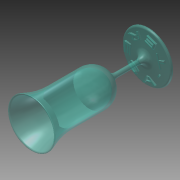
# Autodesk Inventor part: Copas personalizadas
Saved by Autodesk Inventor 2014 (Build 180170000, 170)
## iProperties
Created: 2016-12-26
Part Number: Copas personalizadas
Material: Generic
Document SubType Name: Modeling
Designer: Rubén
Density: 1 g/cm^3
Appearance: Indoor Pool
Author: Rubén
Autodesk Inventor part; units mm, degrees
ref_plane "YZ Plane" through (0, 0, 0) normal (1, 0, 0) x (0, 1, 0)
ref_plane "XZ Plane" through (0, 0, 0) normal (0, 1, 0) x (-1, 0, 0)
ref_plane "XY Plane" through (0, 0, 0) normal (0, 0, 1) x (1, 0, 0)
sketch "Sketch1" plane through (0, 0, 0) normal (1, 0, 0) x (0, 1, 0)
  line L0 (0, 0) -> (0, 70)
  line L1 (0, 70) -> (26, 70)
  line L2 (26, 70) -> (26, 144.9058)
  line L3 (32.0307, 179.1078) -> (36.1508, 190.4275)
  line L4 (38.5, 189.5725) -> (34.38, 178.2528)
  line L5 (28.5, 144.9058) -> (28.5, 67.5)
  line L6 (28.5, 67.5) -> (3.5, 67.5)
  line L7 (3.5, 67.5) -> (3.5, 19.3406)
  line L8 (14.7357, 6.4609) -> (37.4072, 3.3552)
  line L9 (40, 0.3829) -> (40, 0)
  line L10 (40, 0) -> (0, 0)
  line L11 (0, 70) -> (0, 190) construction
  arc A0 (32.0307, 179.1078) -> (26, 144.9058) centre (126, 144.9058) ccw
  arc A1 (34.38, 178.2528) -> (28.5, 144.9058) centre (126, 144.9058) ccw
  line L12 (37.3254, 190) -> (0, 190) construction
  arc A2 (3.5, 19.3406) -> (14.7357, 6.4609) centre (16.5, 19.3406) ccw
  arc A3 (40, 0.3829) -> (37.4072, 3.3552) centre (37, 0.3829) ccw
  line L13 (26, 70) -> (26, 67.5) construction
  line L14 (36.1508, 190.4275) -> (38.5, 189.5725)
  point P0 (26, 162.5385)
  point P1 (28.5, 162.0977)
  point P2 (3.5, 8)
  point P3 (40, 3)
  dimension "d2" = 3
  dimension "d4" = 70
  dimension "d5" = 40
  dimension "d6" = 8
  dimension "d7" = 3.5
  dimension "d10" = 100
  dimension "d14" = 13
  dimension "d15" = 3
  dimension "d26" = 2.5
  dimension "d27" = 10
  dimension "d28" = 26
  dimension "d29" = 160
  dimension "d30" = 190
  constraints: 30 end point, 9 point on line, 8 point on circle, 8 tangent, 5 parallel, 5 perpendicular, 4 centre point, 1 coincident, 1 equal length, 1 horizontal, 1 midpoint, 1 vertical
  measures "d2" distance of point (40, 3) L9.end
  measures "d4" distance of L0.start L0.end
  measures "d5" distance of L9.end L0.start
  measures "d6" distance from line of L10 point (3.5, 8)
  measures "d7" distance between parallel lines of L7 L0
  measures "d10" radius of A0
  measures "d14" radius of A2
  measures "d15" radius of A3
  measures "d26" distance of L1.end L13.end
  measures "d27" distance from line of L5 L4.start
  measures "d28" distance of L0.end L1.end
  measures "d29" angle of L5 L4
  measures "d30" distance between parallel lines of L10 L12
revolve "Revolution1" add sketch "Sketch1" angle 360 about axis through (0, 0, 0) along (0, 0, 1)
fillet "Fillet1" radius 2 2 edges at (0, -36.1508, 190.4275) (0, -38.5, 189.5725)
fillet "Fillet2" radius 26 1 edges at (0, -26, 70)
fillet "Fillet3" radius 15 1 edges at (0, -3.5, 67.5)
fillet "Fillet4" radius 28 1 edges at (0, -28.5, 67.5)
sketch "Sketch2" plane through (0, 0, 0) normal (0, 0, -1) x (-1, 0, 0)
  circle A0 centre (0, 0) radius 40 projected
  constraints: 1 other
extrude "Antonio" [suppressed]
sketch "Sketch3" plane through (0, 0, 0) normal (0, 0, -1) x (-1, 0, 0)
  circle A0 centre (0, 0) radius 40
  line L0 (-32.0557, 8.0153) -> (-23.6218, 5.4451)
  line L1 (-23.6218, 5.4451) -> (-26.0692, -2.5857)
  line L2 (-26.0692, -2.5857) -> (-24.9374, -2.9306)
  line L3 (-24.9374, -2.9306) -> (-19.0741, 16.3092)
  line L4 (-19.0741, 16.3092) -> (-20.2059, 16.6541)
  line L5 (-20.2059, 16.6541) -> (-22.6532, 8.6233)
  line L6 (-22.6532, 8.6233) -> (-31.0872, 11.1935)
  line L7 (-31.0872, 11.1935) -> (-32.0557, 8.0153)
  line L8 (-18.1111, 28.4868) -> (-14.6428, 19.1075)
  line L9 (-14.6428, 19.1075) -> (0.0114, 24.5263)
  line L10 (0.0114, 24.5263) -> (-0.399, 25.636)
  line L11 (-0.399, 25.636) -> (-11.9369, 21.3695)
  line L12 (-11.9369, 21.3695) -> (-12.8869, 23.9386)
  line L13 (-12.8869, 23.9386) -> (-2.1394, 27.9128)
  line L14 (-2.1394, 27.9128) -> (-2.5498, 29.0225)
  line L15 (-2.5498, 29.0225) -> (-13.2972, 25.0483)
  line L16 (-13.2972, 25.0483) -> (-14.5845, 28.5294)
  line L17 (-14.5845, 28.5294) -> (-3.0466, 32.7959)
  line L18 (-3.0466, 32.7959) -> (-3.4569, 33.9056)
  line L19 (-3.4569, 33.9056) -> (-18.1111, 28.4868)
  line L20 (27.5444, 21.3586) -> (23.9465, 23.7338)
  line L21 (23.9465, 23.7338) -> (15.1402, 24.7797)
  line L22 (15.1402, 24.7797) -> (11.9752, 26.8691)
  line L23 (11.9752, 26.8691) -> (14.1673, 30.1897)
  line L24 (14.1673, 30.1897) -> (11.3945, 32.0202)
  line L25 (11.3945, 32.0202) -> (5.8851, 23.6748)
  line L26 (5.8851, 23.6748) -> (11.2616, 20.1254)
  spline S0 degree 2 poles (11.2616, 20.1254) (13.0538, 18.9422) (15.5844, 17.495) (16.8607, 17.0602) knots 0 0 0 1 2 2 2
  spline S1 degree 2 poles (16.8607, 17.0602) (18.1438, 16.621) (20.0001, 16.6675) (20.4332, 17.3235) knots 0 0 0 1 2 2 2
  spline S2 degree 2 poles (20.4332, 17.3235) (21.0359, 18.2365) (19.5265, 21.01) (17.7211, 22.6291) knots 0 0 0 1 2 2 2
  line L27 (17.7211, 22.6291) -> (27.5444, 21.3586)
  spline S3 degree 2 poles (17.5899, 19.3268) (17.3488, 18.9616) (16.3358, 18.8244) (15.539, 19.0883) knots 0 0 0 1 2 2 2
  spline S4 degree 2 poles (15.539, 19.0883) (14.8479, 19.3212) (13.2008, 20.224) (12.0376, 20.992) knots 0 0 0 1 2 2 2
  line L28 (12.0376, 20.992) -> (9.2919, 22.8046)
  line L29 (9.2919, 22.8046) -> (11.3635, 25.9426)
  line L30 (11.3635, 25.9426) -> (13.7981, 24.3353)
  spline S5 degree 2 poles (13.7981, 24.3353) (14.9884, 23.5495) (16.7839, 22.1214) (17.2793, 21.4157) knots 0 0 0 1 2 2 2
  spline S6 degree 2 poles (17.2793, 21.4157) (17.7294, 20.7884) (17.8757, 19.7596) (17.5899, 19.3268) knots 0 0 0 1 2 2 2
  line L31 (32.6068, 8.7352) -> (22.6192, 8.2391)
  line L32 (22.6192, 8.2391) -> (23.3942, -7.3656)
  line L33 (23.3942, -7.3656) -> (24.5759, -7.3069)
  line L34 (24.5759, -7.3069) -> (23.9656, 4.9794)
  line L35 (23.9656, 4.9794) -> (26.7013, 5.1152)
  line L36 (26.7013, 5.1152) -> (27.2697, -6.3293)
  line L37 (27.2697, -6.3293) -> (28.4514, -6.2706)
  line L38 (28.4514, -6.2706) -> (27.883, 5.1739)
  line L39 (27.883, 5.1739) -> (31.59, 5.358)
  line L40 (31.59, 5.358) -> (32.2002, -6.9283)
  line L41 (32.2002, -6.9283) -> (33.3819, -6.8696)
  line L42 (33.3819, -6.8696) -> (32.6068, 8.7352)
  spline S7 degree 2 poles (21.7616, -25.0447) (23.8152, -23.2691) (26.4056, -20.4294) (27.4625, -19.0871) knots 0 0 0 1 2 2 2
  line L43 (27.4625, -19.0871) -> (26.3707, -17.8243)
  line L44 (26.3707, -17.8243) -> (26.1929, -17.978)
  spline S8 degree 2 poles (26.1929, -17.978) (25.3513, -19.5198) (22.6457, -22.7591) (21.1868, -24.0205) knots 0 0 0 1 2 2 2
  spline S9 degree 2 poles (21.1868, -24.0205) (19.1025, -25.8226) (16.3703, -26.9744) (15.8774, -26.4043) knots 0 0 0 1 2 2 2
  spline S10 degree 2 poles (15.8774, -26.4043) (15.4852, -25.9507) (16.1132, -24.4221) (17.2112, -23.2263) knots 0 0 0 1 2 2 2
  spline S11 degree 2 poles (17.2112, -23.2263) (18.003, -22.3703) (19.3331, -20.9846) (20.3289, -19.9308) knots 0 0 0 1 2 2 2
  spline S12 degree 2 poles (20.3289, -19.9308) (21.2196, -18.9785) (22.5002, -17.3249) (22.8775, -16.5595) knots 0 0 0 1 2 2 2
  spline S13 degree 2 poles (22.8775, -16.5595) (23.2425, -15.8046) (23.3093, -14.5685) (22.9276, -14.1271) knots 0 0 0 1 2 2 2
  spline S14 degree 2 poles (22.9276, -14.1271) (22.1326, -13.2076) (17.4767, -15.0586) (14.6936, -17.4649) knots 0 0 0 1 2 2 2
  spline S15 degree 2 poles (14.6936, -17.4649) (13.106, -18.8377) (10.4912, -21.5377) (9.4903, -22.8209) knots 0 0 0 1 2 2 2
  line L45 (9.4903, -22.8209) -> (10.5291, -24.0224)
  line L46 (10.5291, -24.0224) -> (10.7192, -23.8581)
  spline S16 degree 2 poles (10.7192, -23.8581) (11.3341, -22.748) (13.7299, -19.8194) (15.2808, -18.4785) knots 0 0 0 1 2 2 2
  spline S17 degree 2 poles (15.2808, -18.4785) (17.034, -16.9626) (19.7589, -15.7528) (20.22, -16.2861) knots 0 0 0 1 2 2 2
  spline S18 degree 2 poles (20.22, -16.2861) (20.6334, -16.7643) (19.8574, -18.4315) (18.7611, -19.6044) knots 0 0 0 1 2 2 2
  spline S19 degree 2 poles (18.7611, -19.6044) (18.0384, -20.3793) (15.9182, -22.5981) (15.2314, -23.3526) knots 0 0 0 1 2 2 2
  spline S20 degree 2 poles (15.2314, -23.3526) (13.4826, -25.2825) (12.5125, -27.8032) (13.1221, -28.5081) knots 0 0 0 1 2 2 2
  spline S21 degree 2 poles (13.1221, -28.5081) (13.509, -28.9556) (15.1521, -29.0347) (16.2272, -28.6301) knots 0 0 0 1 2 2 2
  spline S22 degree 2 poles (16.2272, -28.6301) (17.4268, -28.1714) (20.0329, -26.5394) (21.7616, -25.0447) knots 0 0 0 1 2 2 2
  line L47 (3.2693, -34.521) -> (-2.7998, -22.9367)
  line L48 (-2.7998, -22.9367) -> (-6.8035, -22.051)
  line L49 (-6.8035, -22.051) -> (-17.1923, -29.9946)
  line L50 (-17.1923, -29.9946) -> (-13.7662, -30.7525)
  line L51 (-13.7662, -30.7525) -> (-10.9469, -28.5128)
  line L52 (-10.9469, -28.5128) -> (-1.626, -30.5747)
  line L53 (-1.626, -30.5747) -> (-0.0144, -33.7946)
  line L54 (-0.0144, -33.7946) -> (3.2693, -34.521)
  line L55 (-9.7998, -27.6046) -> (-5.0148, -23.8327)
  line L56 (-5.0148, -23.8327) -> (-2.2751, -29.2692)
  line L57 (-2.2751, -29.2692) -> (-9.7998, -27.6046)
  line L58 (-24.7506, -11.9445) -> (-22.7476, -15.42)
  line L59 (-22.7476, -15.42) -> (-21.0906, -14.465)
  line L60 (-21.0906, -14.465) -> (-23.0936, -10.9895)
  line L61 (-23.0936, -10.9895) -> (-24.7506, -11.9445)
  constraints: 1 centre point, 1 other
extrude "Teresa" add sketch "Sketch3" against normal blind 7 contours L7 L6 L5 L4 L3 L2 L1 L0 | L19 L18 L17 L16 L15 L14 L13 L12 L11 L10 L9 L8 | L27 S2 S1 S0 L26 L25 L24 L23 L22 L21 L20 | L42 L41 L40 L39 L38 L37 L36 L35 L34 L33 L32 L31 | S22 S21 S20 S19 S18 S17 S16 L46 L45 S15 S14 S13 S12 S11 S10 S9 S8 L44 L43 S7 | L54 L53 L52 L51 L50 L49 L48 L47 | L61 L60 L59 L58
body "Solid1"
